Autodesk Inventor part; units mm, degrees
(part 2 of 3)
sketch "Эскиз8" plane through (0, 0, 2) normal (0, 0, 1) x (1, 0, 0)
  line L0 (83.7862, -21.9654) -> (83.7862, -32.3944) projected
  arc A0 (67.4694, -45.8121) -> (83.7862, -32.3944) centre (57.281, -16.7923) ccw projected
  line L1 (67.4694, -45.8121) -> (61.0555, -45.8121) projected
  arc A1 (53.694, -29.0439) -> (61.0555, -45.8121) centre (61.0555, -35.8121) ccw projected
  line L2 (53.694, -29.0439) -> (66.4247, -15.1972) projected
  arc A2 (83.7862, -21.9654) -> (66.4247, -15.1972) centre (73.7862, -21.9654) ccw projected
  arc A3 (-39.8825, -42.108) -> (-23.8797, -30.3072) centre (-32.521, -35.3398) ccw projected
  line L3 (-39.8825, -42.108) -> (-83.4226, 5.249) projected
  arc A4 (-86.0611, 12.0172) -> (-83.4226, 5.249) centre (-76.0611, 12.0172) ccw projected
  line L4 (-86.0611, 12.0172) -> (-86.0611, 12.0731) projected
  arc A5 (-70.312, 20.2554) -> (-86.0611, 12.0731) centre (-76.0611, 12.0731) ccw projected
  arc A6 (-23.8797, -30.3072) -> (-70.312, 20.2554) centre (-162.6046, -111.0994) ccw projected
  arc A7 (-180.9948, -7.5859) -> (-176.4785, -21.5706) centre (-134.5611, -0.3121) ccw projected
  arc A8 (-176.055, -1.8121) -> (-180.9948, -7.5859) centre (-176.055, -6.8121) ccw projected
  line L5 (-176.055, -1.8121) -> (-162.3245, -1.8121) projected
  arc A9 (-155.2534, -18.8832) -> (-162.3245, -1.8121) centre (-162.3245, -11.8121) ccw projected
  line L6 (-155.2534, -18.8832) -> (-160.4889, -24.1186) projected
  arc A10 (-176.4785, -21.5706) -> (-160.4889, -24.1186) centre (-167.5599, -17.0475) ccw projected
  arc A11 (139.56, -46.7458) -> (153.5447, -42.2296) centre (132.2862, -0.3121) ccw projected
  arc A12 (133.7862, -41.8061) -> (139.56, -46.7458) centre (138.7862, -41.8061) ccw projected
  line L7 (133.7862, -41.8061) -> (133.7862, -28.0756) projected
  arc A13 (150.8573, -21.0045) -> (133.7862, -28.0756) centre (143.7862, -28.0756) ccw projected
  line L8 (150.8573, -21.0045) -> (156.0927, -26.2399) projected
  arc A14 (153.5447, -42.2296) -> (156.0927, -26.2399) centre (149.0216, -33.311) ccw projected
  line L9 (-162.7567, 1.1879) -> (-176.5611, 1.1879) projected
  arc A15 (-181.5611, 6.1879) -> (-176.5611, 1.1879) centre (-176.5611, 6.1879) ccw projected
  line L10 (-181.5611, 6.1879) -> (-181.5611, 31.7702) projected
  arc A16 (-173.2978, 35.5585) -> (-181.5611, 31.7702) centre (-176.5611, 31.7702) ccw projected
  arc A17 (-155.2866, 17.836) -> (-173.2978, 35.5585) centre (-297.8894, -109.0766) ccw projected
  arc A18 (-162.7567, 1.1879) -> (-155.2866, 17.836) centre (-162.7567, 11.1879) ccw projected
  line L11 (81.1477, 5.249) -> (37.6077, -42.108) projected
  arc A19 (21.6048, -30.3072) -> (37.6077, -42.108) centre (30.2462, -35.3398) ccw projected
  arc A20 (68.0372, 20.2554) -> (21.6048, -30.3072) centre (160.3298, -111.0994) ccw projected
  arc A21 (83.7862, 12.0731) -> (68.0372, 20.2554) centre (73.7862, 12.0731) ccw projected
  line L12 (83.7862, 12.0731) -> (83.7862, 12.0172) projected
  arc A22 (81.1477, 5.249) -> (83.7862, 12.0172) centre (73.7862, 12.0172) ccw projected
  arc A23 (136.3136, 14.1371) -> (128.2552, 14.1361) centre (132.2862, -0.3121) ccw projected
  arc A24 (119.19, 16.0661) -> (128.2552, 14.1361) centre (125.5679, 23.7682) ccw projected
  arc A25 (96.4037, 38.427) -> (119.19, 16.0661) centre (240.0147, 161.9803) ccw projected
  arc A26 (100.194, 46.6879) -> (96.4037, 38.427) centre (100.194, 41.6879) ccw projected
  line L13 (100.194, 46.6879) -> (164.3686, 46.6879) projected
  arc A27 (168.1568, 38.4246) -> (164.3686, 46.6879) centre (164.3686, 41.6879) ccw projected
  arc A28 (145.382, 16.0725) -> (168.1568, 38.4246) centre (23.5217, 163.0162) ccw projected
  arc A29 (136.3136, 14.1371) -> (145.382, 16.0725) centre (138.9985, 23.7699) ccw projected
  line L14 (9.0433, 33.3984) -> (33.8141, 6.4561) projected
  arc A30 (33.8141, -7.0803) -> (33.8141, 6.4561) centre (26.4526, -0.3121) ccw projected
  line L15 (33.8141, -7.0803) -> (9.0433, -34.0226) projected
  arc A31 (0.3626, -30.6385) -> (9.0433, -34.0226) centre (5.3626, -30.6385) ccw projected
  line L16 (0.3626, -30.6385) -> (0.3626, 30.0143) projected
  arc A32 (9.0433, 33.3984) -> (0.3626, 30.0143) centre (5.3626, 30.0143) ccw projected
  arc A33 (-166.6434, 46.6879) -> (-170.4316, 38.4246) centre (-166.6434, 41.6879) ccw projected
  line L17 (-166.6434, 46.6879) -> (-102.4688, 46.6879) projected
  arc A34 (-98.6785, 38.427) -> (-102.4688, 46.6879) centre (-102.4688, 41.6879) ccw projected
  arc A35 (-121.4649, 16.0661) -> (-98.6785, 38.427) centre (-242.2895, 161.9803) ccw projected
  arc A36 (-130.53, 14.1361) -> (-121.4649, 16.0661) centre (-127.8427, 23.7682) ccw projected
  arc A37 (-130.53, 14.1361) -> (-138.5884, 14.1371) centre (-134.5611, -0.3121) ccw projected
  arc A38 (-147.6568, 16.0725) -> (-138.5884, 14.1371) centre (-141.2733, 23.7699) ccw projected
  arc A39 (-170.4316, 38.4246) -> (-147.6568, 16.0725) centre (-25.7966, 163.0162) ccw projected
  line L18 (-68.6995, -15.1972) -> (-55.9689, -29.0439) projected
  arc A40 (-63.3304, -45.8121) -> (-55.9689, -29.0439) centre (-63.3304, -35.8121) ccw projected
  line L19 (-63.3304, -45.8121) -> (-69.7443, -45.8121) projected
  arc A41 (-86.0611, -32.3944) -> (-69.7443, -45.8121) centre (-59.5558, -16.7923) ccw projected
  line L20 (-86.0611, -32.3944) -> (-86.0611, -21.9654) projected
  arc A42 (-68.6995, -15.1972) -> (-86.0611, -21.9654) centre (-76.0611, -21.9654) ccw projected
  line L21 (158.214, -24.1186) -> (152.9786, -18.8832) projected
  arc A43 (160.0497, -1.8121) -> (152.9786, -18.8832) centre (160.0497, -11.8121) ccw projected
  line L22 (160.0497, -1.8121) -> (173.7802, -1.8121) projected
  arc A44 (178.72, -7.5859) -> (173.7802, -1.8121) centre (173.7802, -6.8121) ccw projected
  arc A45 (174.2037, -21.5706) -> (178.72, -7.5859) centre (132.2862, -0.3121) ccw projected
  arc A46 (158.214, -24.1186) -> (174.2037, -21.5706) centre (165.2851, -17.0475) ccw projected
  arc A47 (95.0878, 34.2305) -> (86.7862, 30.4755) centre (91.7862, 30.4755) ccw projected
  arc A48 (115.908, 12.7841) -> (95.0878, 34.2305) centre (-30.0061, -108.0406) ccw projected
  arc A49 (117.838, 3.7189) -> (115.908, 12.7841) centre (108.2059, 6.4063) ccw projected
  arc A50 (117.838, 3.7189) -> (117.837, -4.3395) centre (132.2862, -0.3121) ccw projected
  arc A51 (115.9016, -13.4079) -> (117.837, -4.3395) centre (108.2042, -7.0244) ccw projected
  arc A52 (95.0899, -34.8414) -> (115.9016, -13.4079) centre (-31.0421, 108.4524) ccw projected
  arc A53 (86.7862, -31.0883) -> (95.0899, -34.8414) centre (91.7862, -31.0883) ccw projected
  line L23 (86.7862, -31.0883) -> (86.7862, 30.4755) projected
  arc A54 (174.2862, 1.1879) -> (179.2862, 6.1879) centre (174.2862, 6.1879) ccw projected
  line L24 (174.2862, 1.1879) -> (160.4818, 1.1879) projected
  arc A55 (153.0118, 17.836) -> (160.4818, 1.1879) centre (160.4818, 11.1879) ccw projected
  arc A56 (171.0229, 35.5585) -> (153.0118, 17.836) centre (295.6146, -109.0766) ccw projected
  arc A57 (179.2862, 31.7702) -> (171.0229, 35.5585) centre (174.2862, 31.7702) ccw projected
  line L25 (179.2862, 31.7702) -> (179.2862, 6.1879) projected
  line L26 (-11.3182, -34.0226) -> (-36.0889, -7.0803) projected
  arc A58 (-36.0889, 6.4561) -> (-36.0889, -7.0803) centre (-28.7274, -0.3121) ccw projected
  line L27 (-36.0889, 6.4561) -> (-11.3182, 33.3984) projected
  arc A59 (-2.6374, 30.0143) -> (-11.3182, 33.3984) centre (-7.6374, 30.0143) ccw projected
  line L28 (-2.6374, 30.0143) -> (-2.6374, -30.6385) projected
  arc A60 (-11.3182, -34.0226) -> (-2.6374, -30.6385) centre (-7.6374, -30.6385) ccw projected
  line L29 (-158.3675, -26.2399) -> (-153.1321, -21.0045) projected
  arc A61 (-136.0611, -28.0756) -> (-153.1321, -21.0045) centre (-146.0611, -28.0756) ccw projected
  line L30 (-136.0611, -28.0756) -> (-136.0611, -41.8061) projected
  arc A62 (-141.8349, -46.7458) -> (-136.0611, -41.8061) centre (-141.0611, -41.8061) ccw projected
  arc A63 (-155.8196, -42.2296) -> (-141.8349, -46.7458) centre (-134.5611, -0.3121) ccw projected
  arc A64 (-158.3675, -26.2399) -> (-155.8196, -42.2296) centre (-151.2965, -33.311) ccw projected
  arc A65 (-120.1118, -4.3395) -> (-120.1128, 3.7189) centre (-134.5611, -0.3121) ccw projected
  arc A66 (-118.1829, 12.7841) -> (-120.1128, 3.7189) centre (-110.4807, 6.4063) ccw projected
  arc A67 (-97.3626, 34.2305) -> (-118.1829, 12.7841) centre (27.7313, -108.0406) ccw projected
  arc A68 (-89.0611, 30.4755) -> (-97.3626, 34.2305) centre (-94.0611, 30.4755) ccw projected
  line L31 (-89.0611, 30.4755) -> (-89.0611, -31.0883) projected
  arc A69 (-97.3647, -34.8414) -> (-89.0611, -31.0883) centre (-94.0611, -31.0883) ccw projected
  arc A70 (-118.1765, -13.4079) -> (-97.3647, -34.8414) centre (28.7673, 108.4524) ccw projected
  arc A71 (-120.1118, -4.3395) -> (-118.1765, -13.4079) centre (-110.479, -7.0244) ccw projected
  arc A72 (-102.4787, -47.3121) -> (-98.6905, -39.0488) centre (-102.4787, -42.3121) ccw projected
  line L32 (-102.4787, -47.3121) -> (-128.0611, -47.3121) projected
  arc A73 (-133.0611, -42.3121) -> (-128.0611, -47.3121) centre (-128.0611, -42.3121) ccw projected
  line L33 (-133.0611, -42.3121) -> (-133.0611, -28.5077) projected
  arc A74 (-116.4129, -21.0376) -> (-133.0611, -28.5077) centre (-123.0611, -28.5077) ccw projected
  arc A75 (-98.6905, -39.0488) -> (-116.4129, -21.0376) centre (-243.3255, -163.6405) ccw projected
  arc A76 (-74.1343, 46.6879) -> (-77.8151, 38.3038) centre (-74.1343, 41.6879) ccw projected
  line L34 (-74.1343, 46.6879) -> (-14.5641, 46.6879) projected
  arc A77 (-10.8834, 38.3038) -> (-14.5641, 46.6879) centre (-14.5641, 41.6879) ccw projected
  line L35 (-10.8834, 38.3038) -> (-36.9877, 9.911) projected
  arc A78 (-51.7107, 9.911) -> (-36.9877, 9.911) centre (-44.3492, 16.6792) ccw projected
  line L36 (-51.7107, 9.911) -> (-77.8151, 38.3038) projected
  arc A79 (130.7862, -28.5077) -> (114.1381, -21.0376) centre (120.7862, -28.5077) ccw projected
  line L37 (130.7862, -28.5077) -> (130.7862, -42.3121) projected
  arc A80 (125.7862, -47.3121) -> (130.7862, -42.3121) centre (125.7862, -42.3121) ccw projected
  line L38 (125.7862, -47.3121) -> (100.2039, -47.3121) projected
  arc A81 (96.4156, -39.0488) -> (100.2039, -47.3121) centre (100.2039, -42.3121) ccw projected
  arc A82 (114.1381, -21.0376) -> (96.4156, -39.0488) centre (241.0507, -163.6405) ccw projected
  line L39 (75.5403, 38.3038) -> (49.4359, 9.911) projected
  arc A83 (34.7129, 9.911) -> (49.4359, 9.911) centre (42.0744, 16.6792) ccw projected
  line L40 (34.7129, 9.911) -> (8.6085, 38.3038) projected
  arc A84 (12.2893, 46.6879) -> (8.6085, 38.3038) centre (12.2893, 41.6879) ccw projected
  line L41 (12.2893, 46.6879) -> (71.8595, 46.6879) projected
  arc A85 (75.5403, 38.3038) -> (71.8595, 46.6879) centre (71.8595, 41.6879) ccw projected
  line L42 (179.2862, 51.6879) -> (-181.5611, 51.6879) projected
  arc A86 (-181.5611, 51.6879) -> (-186.5611, 46.6879) centre (-181.5611, 46.6879) ccw projected
  line L43 (-186.5611, 46.6879) -> (-186.5611, -0.3121) projected
  arc A87 (-186.5611, -0.3121) -> (-134.5611, -52.3121) centre (-134.5611, -0.3121) ccw projected
  line L44 (-134.5611, -52.3121) -> (132.2862, -52.3121) projected
  arc A88 (132.2862, -52.3121) -> (184.2862, -0.3121) centre (132.2862, -0.3121) ccw projected
  line L45 (184.2862, -0.3121) -> (184.2862, 46.6879) projected
  arc A89 (184.2862, 46.6879) -> (179.2862, 51.6879) centre (179.2862, 46.6879) ccw projected
  circle A90 centre (85.2862, -47.3121) radius 2.1 projected
  circle A91 centre (179.2862, 46.6879) radius 2.1 projected
  circle A92 centre (85.2862, 46.6879) radius 2.1 projected
  circle A93 centre (-1.1374, 46.6879) radius 2.1 projected
  circle A94 centre (-87.5611, 46.6879) radius 2.1 projected
  circle A95 centre (-181.5611, 46.6879) radius 2.1 projected
  circle A96 centre (-87.5611, -47.3121) radius 2.1 projected
  circle A97 centre (123.2862, -0.3121) radius 2.1 projected
  circle A98 centre (132.2862, 8.6879) radius 2.1 projected
  circle A99 centre (-125.5611, -0.3121) radius 2.1 projected
  circle A100 centre (-134.5611, -9.3121) radius 2.1 projected
  circle A101 centre (-134.5611, 8.6879) radius 2.1 projected
  circle A102 centre (-1.1374, -47.3121) radius 2.1 projected
  circle A103 centre (132.2862, -0.3121) radius 4 projected
  circle A104 centre (132.2862, -9.3121) radius 2.1 projected
  circle A105 centre (141.2862, -0.3121) radius 2.1 projected
  circle A106 centre (-143.5611, -0.3121) radius 2.1 projected
  circle A107 centre (-134.5611, -0.3121) radius 4 projected
  line L46 (132.2862, -47.3121) -> (-134.5611, -47.3121)
  arc A108 (-181.5611, -0.3121) -> (-134.5611, -47.3121) centre (-134.5611, -0.3121) ccw
  line L47 (-181.5611, -0.3121) -> (-181.5611, 46.6879)
  line L48 (-181.5611, 46.6879) -> (179.2862, 46.6879)
  line L49 (179.2862, 46.6879) -> (179.2862, -0.3121)
  arc A109 (132.2862, -47.3121) -> (179.2862, -0.3121) centre (132.2862, -0.3121) ccw
  line L50 (-87.5611, -52.3121) -> (-87.5611, -33.3121)
  line L51 (-87.5611, -33.3121) -> (-207.6837, -33.3121)
  line L52 (-207.6837, -33.3121) -> (179.2862, -33.3121)
  point P0 (0, 0)
  point P1 (-174.7481, -33.3121)
  point P2 (172.4733, -33.3121)
  point P3 (153.3812, -42.3121)
  point P4 (133.8119, -42.3121)
  point P5 (95.2039, -42.3121)
  point P6 (83.2242, -33.3121)
  point P7 (51.3731, -33.3121)
  point P8 (37.4147, -42.3121)
  point P9 (20.4539, -33.3121)
  point P10 (-22.7287, -33.3121)
  point P11 (-39.6895, -42.3121)
  point P12 (-53.6479, -33.3121)
  point P13 (-85.499, -33.3121)
  point P14 (130.7862, -33.3121)
  point P15 (101.5627, -33.3121)
  point P16 (159.0216, -33.3121)
  point P17 (133.7862, -33.3121)
  point P18 (45.6946, -33.3121)
  point P19 (-47.9694, -33.3121)
  dimension "d101" = 19
  constraints: 12 end point, 4 point on circle, 2 centre point, 2 perpendicular, 2 point on line, 8 other
  measures "d101" distance of L50.start L50.end
extrude "Выдавливание6" cut sketch "Эскиз8" against normal blind 2 contours L52 A53 A52 A82 A81 L46 A90 A102 A96 L50 A41 L19 A40 L3 A3 L26 A60 A31 L15 A19 L11 A1 L1 A0 | A0 L1 A1 L52 | L52 A52 A53 | L11 A19 L52 | L52 L37 A80 L38 A81 A82 | L15 A31 L52 | L52 L7 A12 A109 L46 A80 L37 | L38 L46 A109 A11 L52 A88 L44 L50 A96 A102 A90 | L52 A14 A11 A12 L7 | A60 L26 L52 | L52 A109 A14 | A3 L3 L52 | A40 L19 A41 L52 | L44 A87 L51 A108 A63 L46 L32 A96 L50 | A96 L46 A72 A75 L51 A70 A69 L50 | A69 A70 L51 | L32 A73 L33 L51 A75 A72 | L51 A64 A108 | L46 A108 A62 L30 L51 L33 A73 | A64 L51 L30 A62 A63
sketch "Эскиз9" plane through (0, 0, 2) normal (0, 0, 1) x (1, 0, 0)
  arc A0 (-186.5611, -0.3121) -> (-174.7481, -33.3121) centre (-134.5611, -0.3121) ccw projected
  arc A1 (172.4733, -33.3121) -> (184.2862, -0.3121) centre (132.2862, -0.3121) ccw projected
  line L0 (-198, -37.3121) -> (220, -37.3121)
  line L1 (-198, -28.3121) -> (220, -28.3121)
  line L2 (-174.7481, -33.3121) -> (-161.2965, -33.3121) projected
  line L3 (-174.7481, -33.3121) -> (172.4733, -33.3121)
  point P0 (0, 0)
  point P1 (168.8239, -37.3121)
  point P2 (-171.0987, -37.3121)
  point P3 (176.104, -28.3121)
  point P4 (-178.3789, -28.3121)
  dimension "d118" = 9
  constraints: 6 end point, 1 collinear, 1 parallel
  measures "d118" distance between parallel lines of L0 L1
extrude "Выдавливание7" add sketch "Эскиз9" against normal blind 2
fillet "Сопряжение6" radius 3 26 edges at (-174.7481, -33.3121, 1) (172.4733, -33.3121, 1) (-159.9574, -28.3121, 1) (-136.0611, -28.3121, 1) (-133.0592, -28.3121, 1) (-108.683, -28.3121, 1) (-104.4163, -28.3121, 1) (-89.0611, -28.3121, 1) (-86.0611, -28.3121, 1) (-56.6417, -28.3121, 1) (-25.061, -28.3121, 1) (-2.6374, -28.3121, 1) (14.2936, -28.3121, 1) (50.2916, -28.3121, 1) (83.7862, -28.3121, 1) (102.1414, -28.3121, 1) (130.7843, -28.3121, 1) (157.6826, -28.3121, 1) (-52.5665, -28.3121, 1) (-16.5684, -28.3121, 1) (0.3626, -28.3121, 1) (22.7861, -28.3121, 1) (54.3669, -28.3121, 1) (86.7862, -28.3121, 1) (106.4081, -28.3121, 1) (133.7862, -28.3121, 1)
sketch "Эскиз10" plane through (0, 0, 2) normal (0, 0, 1) x (1, 0, 0)
  circle A0 centre (-87.5611, 46.6879) radius 2.1 projected
  circle A1 centre (-1.1374, 46.6879) radius 2.1 projected
  circle A2 centre (85.2862, 46.6879) radius 2.1 projected
  line L0 (179.2862, 51.6879) -> (-181.5611, 51.6879) projected
  line L1 (-1.1374, 51.6879) -> (-1.1374, -33.3121)
  line L2 (171.029, -33.3121) -> (-173.3038, -33.3121) projected
  line L3 (-1.1374, 9.1879) -> (-298, 9.1879)
  line L4 (-298, 9.1879) -> (290, 9.1879)
  circle A3 centre (-87.5611, -28.3121) radius 2.1
  circle A4 centre (-1.1374, -28.3121) radius 2.1
  circle A5 centre (85.2862, -28.3121) radius 2.1
  point P0 (0, 0)
  constraints: 6 end point, 3 centre point, 3 midpoint, 3 symmetric about line, 2 horizontal, 3 other
extrude "Выдавливание8" cut sketch "Эскиз10" against normal blind 2 contours A4 L1 | L1 A4 | A3 | A5
sketch "Эскиз11" plane through (0, 0, 2) normal (0, 0, 1) x (1, 0, 0)
  arc A0 (171.029, -33.3121) -> (173.401, -32.1488) centre (171.029, -30.3121) ccw projected
  arc A1 (173.401, -32.1488) -> (184.2862, -0.3121) centre (132.2862, -0.3121) ccw projected
  line L0 (184.2862, -0.3121) -> (184.2862, 46.6879) projected
  arc A2 (184.2862, 46.6879) -> (179.2862, 51.6879) centre (179.2862, 46.6879) ccw projected
  line L1 (179.2862, 51.6879) -> (-181.5611, 51.6879) projected
  arc A3 (-181.5611, 51.6879) -> (-186.5611, 46.6879) centre (-181.5611, 46.6879) ccw projected
  line L2 (-186.5611, 46.6879) -> (-186.5611, -0.3121) projected
  arc A4 (-186.5611, -0.3121) -> (-175.6758, -32.1488) centre (-134.5611, -0.3121) ccw projected
  arc A5 (-175.6758, -32.1488) -> (-173.3038, -33.3121) centre (-173.3038, -30.3121) ccw projected
  line L3 (-173.3038, -33.3121) -> (171.029, -33.3121) projected
  line L4 (-155.3184, -23.1908) -> (-153.1321, -21.0045) projected
  arc A6 (-136.8733, -24.1278) -> (-153.1321, -21.0045) centre (-146.0611, -28.0756) ccw projected
  arc A7 (68.0372, 20.2554) -> (25.6837, -23.6784) centre (160.3298, -111.0994) ccw projected
  arc A8 (83.7862, 12.0731) -> (68.0372, 20.2554) centre (73.7862, 12.0731) ccw projected
  line L5 (83.7862, 12.0731) -> (83.7862, 12.0172) projected
  arc A9 (81.1477, 5.249) -> (83.7862, 12.0172) centre (73.7862, 12.0172) ccw projected
  line L6 (81.1477, 5.249) -> (51.183, -27.3426) projected
  line L7 (-53.4579, -27.3426) -> (-83.4226, 5.249) projected
  arc A10 (-86.0611, 12.0172) -> (-83.4226, 5.249) centre (-76.0611, 12.0172) ccw projected
  line L8 (-86.0611, 12.0172) -> (-86.0611, 12.0731) projected
  arc A11 (-70.312, 20.2554) -> (-86.0611, 12.0731) centre (-76.0611, 12.0731) ccw projected
  arc A12 (-27.9585, -23.6784) -> (-70.312, 20.2554) centre (-162.6046, -111.0994) ccw projected
  arc A13 (114.1381, -21.0376) -> (111.8541, -23.1036) centre (241.0507, -163.6405) ccw projected
  arc A14 (129.6834, -23.9426) -> (114.1381, -21.0376) centre (120.7862, -28.5077) ccw projected
  arc A15 (-68.6995, -15.1972) -> (-86.0611, -21.9654) centre (-76.0611, -21.9654) ccw projected
  line L9 (-68.6995, -15.1972) -> (-61.2667, -23.2817) projected
  line L10 (58.9919, -23.2817) -> (66.4247, -15.1972) projected
  arc A16 (83.7862, -21.9654) -> (66.4247, -15.1972) centre (73.7862, -21.9654) ccw projected
  line L11 (83.7862, -21.9654) -> (83.7862, -25.3121) projected
  arc A17 (-116.4129, -21.0376) -> (-131.9582, -23.9426) centre (-123.0611, -28.5077) ccw projected
  arc A18 (-114.1289, -23.1036) -> (-116.4129, -21.0376) centre (-243.3255, -163.6405) ccw projected
  arc A19 (150.8573, -21.0045) -> (134.5985, -24.1278) centre (143.7862, -28.0756) ccw projected
  line L12 (150.8573, -21.0045) -> (153.0436, -23.1908) projected
  circle A20 centre (-134.5611, -0.3121) radius 4 projected
  circle A21 centre (-143.5611, -0.3121) radius 2.1 projected
  circle A22 centre (141.2862, -0.3121) radius 2.1 projected
  circle A23 centre (132.2862, -9.3121) radius 2.1 projected
  circle A24 centre (132.2862, -0.3121) radius 4 projected
  circle A25 centre (-134.5611, 8.6879) radius 2.1 projected
  circle A26 centre (-134.5611, -9.3121) radius 2.1 projected
  circle A27 centre (-125.5611, -0.3121) radius 2.1 projected
  circle A28 centre (132.2862, 8.6879) radius 2.1 projected
  circle A29 centre (123.2862, -0.3121) radius 2.1 projected
  circle A30 centre (-181.5611, 46.6879) radius 2.1 projected
  circle A31 centre (-87.5611, 46.6879) radius 2.1 projected
  circle A32 centre (-1.1374, 46.6879) radius 2.1 projected
  circle A33 centre (85.2862, 46.6879) radius 2.1 projected
  circle A34 centre (179.2862, 46.6879) radius 2.1 projected
  line L13 (75.5403, 38.3038) -> (49.4359, 9.911) projected
  arc A35 (34.7129, 9.911) -> (49.4359, 9.911) centre (42.0744, 16.6792) ccw projected
  line L14 (34.7129, 9.911) -> (8.6085, 38.3038) projected
  arc A36 (12.2893, 46.6879) -> (8.6085, 38.3038) centre (12.2893, 41.6879) ccw projected
  line L15 (12.2893, 46.6879) -> (71.8595, 46.6879) projected
  arc A37 (75.5403, 38.3038) -> (71.8595, 46.6879) centre (71.8595, 41.6879) ccw projected
  arc A38 (-74.1343, 46.6879) -> (-77.8151, 38.3038) centre (-74.1343, 41.6879) ccw projected
  line L16 (-74.1343, 46.6879) -> (-14.5641, 46.6879) projected
  arc A39 (-10.8834, 38.3038) -> (-14.5641, 46.6879) centre (-14.5641, 41.6879) ccw projected
  line L17 (-10.8834, 38.3038) -> (-36.9877, 9.911) projected
  arc A40 (-51.7107, 9.911) -> (-36.9877, 9.911) centre (-44.3492, 16.6792) ccw projected
  line L18 (-51.7107, 9.911) -> (-77.8151, 38.3038) projected
  arc A41 (-120.1118, -4.3395) -> (-120.1128, 3.7189) centre (-134.5611, -0.3121) ccw projected
  arc A42 (-118.1829, 12.7841) -> (-120.1128, 3.7189) centre (-110.4807, 6.4063) ccw projected
  arc A43 (-97.3626, 34.2305) -> (-118.1829, 12.7841) centre (27.7313, -108.0406) ccw projected
  arc A44 (-89.0611, 30.4755) -> (-97.3626, 34.2305) centre (-94.0611, 30.4755) ccw projected
  line L19 (-89.0611, 30.4755) -> (-89.0611, -25.3121) projected
  arc A45 (-118.1765, -13.4079) -> (-105.2981, -27.4478) centre (28.7673, 108.4524) ccw projected
  arc A46 (-120.1118, -4.3395) -> (-118.1765, -13.4079) centre (-110.479, -7.0244) ccw projected
  line L20 (-17.4598, -27.3426) -> (-36.0889, -7.0803) projected
  arc A47 (-36.0889, 6.4561) -> (-36.0889, -7.0803) centre (-28.7274, -0.3121) ccw projected
  line L21 (-36.0889, 6.4561) -> (-11.3182, 33.3984) projected
  arc A48 (-2.6374, 30.0143) -> (-11.3182, 33.3984) centre (-7.6374, 30.0143) ccw projected
  line L22 (-2.6374, 30.0143) -> (-2.6374, -25.3121) projected
  arc A49 (174.2862, 1.1879) -> (179.2862, 6.1879) centre (174.2862, 6.1879) ccw projected
  line L23 (174.2862, 1.1879) -> (160.4818, 1.1879) projected
  arc A50 (153.0118, 17.836) -> (160.4818, 1.1879) centre (160.4818, 11.1879) ccw projected
  arc A51 (171.0229, 35.5585) -> (153.0118, 17.836) centre (295.6146, -109.0766) ccw projected
  arc A52 (179.2862, 31.7702) -> (171.0229, 35.5585) centre (174.2862, 31.7702) ccw projected
  line L24 (179.2862, 31.7702) -> (179.2862, 6.1879) projected
  arc A53 (95.0878, 34.2305) -> (86.7862, 30.4755) centre (91.7862, 30.4755) ccw projected
  arc A54 (115.908, 12.7841) -> (95.0878, 34.2305) centre (-30.0061, -108.0406) ccw projected
  arc A55 (117.838, 3.7189) -> (115.908, 12.7841) centre (108.2059, 6.4063) ccw projected
  arc A56 (117.838, 3.7189) -> (117.837, -4.3395) centre (132.2862, -0.3121) ccw projected
  arc A57 (115.9016, -13.4079) -> (117.837, -4.3395) centre (108.2042, -7.0244) ccw projected
  arc A58 (103.0232, -27.4478) -> (115.9016, -13.4079) centre (-31.0421, 108.4524) ccw projected
  line L25 (86.7862, -25.3121) -> (86.7862, 30.4755) projected
  line L26 (158.214, -24.1186) -> (152.9786, -18.8832) projected
  arc A59 (160.0497, -1.8121) -> (152.9786, -18.8832) centre (160.0497, -11.8121) ccw projected
  line L27 (160.0497, -1.8121) -> (173.7802, -1.8121) projected
  arc A60 (178.72, -7.5859) -> (173.7802, -1.8121) centre (173.7802, -6.8121) ccw projected
  arc A61 (174.2037, -21.5706) -> (178.72, -7.5859) centre (132.2862, -0.3121) ccw projected
  arc A62 (158.214, -24.1186) -> (174.2037, -21.5706) centre (165.2851, -17.0475) ccw projected
  arc A63 (-166.6434, 46.6879) -> (-170.4316, 38.4246) centre (-166.6434, 41.6879) ccw projected
  line L28 (-166.6434, 46.6879) -> (-102.4688, 46.6879) projected
  arc A64 (-98.6785, 38.427) -> (-102.4688, 46.6879) centre (-102.4688, 41.6879) ccw projected
  arc A65 (-121.4649, 16.0661) -> (-98.6785, 38.427) centre (-242.2895, 161.9803) ccw projected
  arc A66 (-130.53, 14.1361) -> (-121.4649, 16.0661) centre (-127.8427, 23.7682) ccw projected
  arc A67 (-130.53, 14.1361) -> (-138.5884, 14.1371) centre (-134.5611, -0.3121) ccw projected
  arc A68 (-147.6568, 16.0725) -> (-138.5884, 14.1371) centre (-141.2733, 23.7699) ccw projected
  arc A69 (-170.4316, 38.4246) -> (-147.6568, 16.0725) centre (-25.7966, 163.0162) ccw projected
  line L29 (9.0433, 33.3984) -> (33.8141, 6.4561) projected
  arc A70 (33.8141, -7.0803) -> (33.8141, 6.4561) centre (26.4526, -0.3121) ccw projected
  line L30 (33.8141, -7.0803) -> (15.185, -27.3426) projected
  line L31 (0.3626, -25.3121) -> (0.3626, 30.0143) projected
  arc A71 (9.0433, 33.3984) -> (0.3626, 30.0143) centre (5.3626, 30.0143) ccw projected
  arc A72 (136.3136, 14.1371) -> (128.2552, 14.1361) centre (132.2862, -0.3121) ccw projected
  arc A73 (119.19, 16.0661) -> (128.2552, 14.1361) centre (125.5679, 23.7682) ccw projected
  arc A74 (96.4037, 38.427) -> (119.19, 16.0661) centre (240.0147, 161.9803) ccw projected
  arc A75 (100.194, 46.6879) -> (96.4037, 38.427) centre (100.194, 41.6879) ccw projected
  line L32 (100.194, 46.6879) -> (164.3686, 46.6879) projected
  arc A76 (168.1568, 38.4246) -> (164.3686, 46.6879) centre (164.3686, 41.6879) ccw projected
  arc A77 (145.382, 16.0725) -> (168.1568, 38.4246) centre (23.5217, 163.0162) ccw projected
  arc A78 (136.3136, 14.1371) -> (145.382, 16.0725) centre (138.9985, 23.7699) ccw projected
  line L33 (-162.7567, 1.1879) -> (-176.5611, 1.1879) projected
  arc A79 (-181.5611, 6.1879) -> (-176.5611, 1.1879) centre (-176.5611, 6.1879) ccw projected
  line L34 (-181.5611, 6.1879) -> (-181.5611, 31.7702) projected
  arc A80 (-173.2978, 35.5585) -> (-181.5611, 31.7702) centre (-176.5611, 31.7702) ccw projected
  arc A81 (-155.2866, 17.836) -> (-173.2978, 35.5585) centre (-297.8894, -109.0766) ccw projected
  arc A82 (-162.7567, 1.1879) -> (-155.2866, 17.836) centre (-162.7567, 11.1879) ccw projected
  arc A83 (-180.9948, -7.5859) -> (-176.4785, -21.5706) centre (-134.5611, -0.3121) ccw projected
  arc A84 (-176.055, -1.8121) -> (-180.9948, -7.5859) centre (-176.055, -6.8121) ccw projected
  line L35 (-176.055, -1.8121) -> (-162.3245, -1.8121) projected
  arc A85 (-155.2534, -18.8832) -> (-162.3245, -1.8121) centre (-162.3245, -11.8121) ccw projected
  line L36 (-155.2534, -18.8832) -> (-160.4889, -24.1186) projected
  arc A86 (-176.4785, -21.5706) -> (-160.4889, -24.1186) centre (-167.5599, -17.0475) ccw projected
  circle A87 centre (-87.5611, -28.3121) radius 5
  circle A88 centre (-1.1374, -28.3121) radius 5
  circle A89 centre (85.2862, -28.3121) radius 5
  line L37 (-1.1374, 46.6879) -> (-1.1374, -28.3121)
  line L38 (-1.1374, 9.1879) -> (8.8626, 9.1879)
  line L39 (-2.6374, -25.3121) -> (-2.6374, 30.0143) projected
  line L40 (-1.1374, 9.1879) -> (8.8626, 9.1879) construction
  arc A90 (71.8595, -28.3121) -> (83.7862, -21.9654) centre (72.2556, -14.6768) ccw
  arc A91 (-86.0611, -21.9654) -> (-74.1343, -28.3121) centre (-74.5305, -14.6768) ccw
  circle A92 centre (85.2862, -28.3121) radius 2.1 projected
  circle A93 centre (-87.5611, -28.3121) radius 2.1 projected
  line L41 (-86.0611, -25.3121) -> (-86.0611, -21.9654) projected
  circle A94 centre (-1.1374, -28.3121) radius 2.1 projected
  line L42 (-92.0611, -28.3121) -> (-103.1912, -28.3121) projected
  line L43 (-63.4752, -28.3121) -> (-83.0611, -28.3121) projected
  line L44 (-5.6374, -28.3121) -> (-15.2513, -28.3121) projected
  line L45 (100.9164, -28.3121) -> (89.7862, -28.3121) projected
  line L46 (12.9765, -28.3121) -> (3.3626, -28.3121) projected
  line L47 (80.7862, -28.3121) -> (61.2003, -28.3121) projected
  line L48 (127.0142, -28.3121) -> (113.8844, -28.3121) projected
  line L49 (48.9746, -28.3121) -> (28.1999, -28.3121) projected
  line L50 (150.9223, -28.3121) -> (137.3548, -28.3121) projected
  line L51 (-30.4747, -28.3121) -> (-51.2494, -28.3121) projected
  line L52 (-139.6296, -28.3121) -> (-153.1971, -28.3121) projected
  line L53 (-116.1593, -28.3121) -> (-129.2891, -28.3121) projected
  arc A95 (-139.6296, -28.3121) -> (-136.8733, -24.1278) centre (-139.6296, -25.3121) ccw projected
  arc A96 (-155.3184, -23.1908) -> (-153.1971, -28.3121) centre (-153.1971, -25.3121) ccw projected
  arc A97 (100.9164, -28.3121) -> (103.0232, -27.4478) centre (100.9164, -25.3121) ccw projected
  arc A98 (127.0142, -28.3121) -> (129.6834, -23.9426) centre (127.0142, -25.3121) ccw projected
  arc A99 (80.7862, -28.3121) -> (83.7862, -25.3121) centre (80.7862, -25.3121) ccw projected
  arc A100 (48.9746, -28.3121) -> (51.183, -27.3426) centre (48.9746, -25.3121) ccw projected
  arc A101 (150.9223, -28.3121) -> (153.0436, -23.1908) centre (150.9223, -25.3121) ccw projected
  arc A102 (0.3626, -25.3121) -> (3.3626, -28.3121) centre (3.3626, -25.3121) ccw projected
  arc A103 (12.9765, -28.3121) -> (15.185, -27.3426) centre (12.9765, -25.3121) ccw projected
  arc A104 (-17.4598, -27.3426) -> (-15.2513, -28.3121) centre (-15.2513, -25.3121) ccw projected
  arc A105 (-5.6374, -28.3121) -> (-2.6374, -25.3121) centre (-5.6374, -25.3121) ccw projected
  arc A106 (-53.4579, -27.3426) -> (-51.2494, -28.3121) centre (-51.2494, -25.3121) ccw projected
  arc A107 (-30.4747, -28.3121) -> (-27.9585, -23.6784) centre (-30.4747, -25.3121) ccw projected
  arc A108 (-86.0611, -25.3121) -> (-83.0611, -28.3121) centre (-83.0611, -25.3121) ccw projected
  arc A109 (-63.4752, -28.3121) -> (-61.2667, -23.2817) centre (-63.4752, -25.3121) ccw projected
  arc A110 (-116.1593, -28.3121) -> (-114.1289, -23.1036) centre (-116.1593, -25.3121) ccw projected
  arc A111 (-131.9582, -23.9426) -> (-129.2891, -28.3121) centre (-129.2891, -25.3121) ccw projected
  arc A112 (-105.2981, -27.4478) -> (-103.1912, -28.3121) centre (-103.1912, -25.3121) ccw projected
  arc A113 (-92.0611, -28.3121) -> (-89.0611, -25.3121) centre (-92.0611, -25.3121) ccw projected
  arc A114 (86.7862, -25.3121) -> (89.7862, -28.3121) centre (89.7862, -25.3121) ccw projected
  arc A115 (111.8541, -23.1036) -> (113.8844, -28.3121) centre (113.8844, -25.3121) ccw projected
  arc A116 (58.9919, -23.2817) -> (61.2003, -28.3121) centre (61.2003, -25.3121) ccw projected
  arc A117 (25.6837, -23.6784) -> (28.1999, -28.3121) centre (28.1999, -25.3121) ccw projected
  arc A118 (134.5985, -24.1278) -> (137.3548, -28.3121) centre (137.3548, -25.3121) ccw projected
  arc A119 (86.7862, -12.0997) -> (100.194, -28.3121) centre (105.7085, -10.1012) ccw
  arc A120 (0.3626, -11.6385) -> (12.2893, -28.3121) centre (15.857, -13.1577) ccw
  arc A121 (-102.4688, -28.3121) -> (-89.0611, -12.0997) centre (-107.9833, -10.1012) ccw
  arc A122 (-14.5641, -28.3121) -> (-2.6374, -11.6385) centre (-18.1319, -13.1577) ccw
  point P0 (0, 0)
  point P1 (-2.6374, -30.6385)
  point P2 (-2.6374, -26.8424)
  point P3 (-2.6374, -26.8424)
  point P4 (72.6518, -28.3121)
  point P5 (100.194, -28.3121)
  point P6 (86.7862, -12.0997)
  point P7 (-2.6374, -14.6768)
  point P8 (-14.5641, -28.3121)
  point P9 (12.2893, -28.3121)
  point P10 (0.3626, -14.6768)
  point P11 (-74.9266, -28.3121)
  point P12 (-89.0611, -12.0997)
  point P13 (-102.4688, -28.3121)
  dimension "d110" = 10
  dimension "d111" = 10
  dimension "d112" = 10
  dimension "d113" = 10
  dimension "d114" = 0
  constraints: 13 symmetric about line, 12 point on circle, 9 centre point, 6 end point, 2 perpendicular, 1 collinear, 1 horizontal, 1 midpoint, 3 other
  measures "d110" diameter of A87
  measures "d111" diameter of A88
  measures "d112" diameter of A89
  measures "d113" distance of L38.start L38.end
  measures "d114" distance between parallel lines of L38 L40
extrude "Выдавливание9" add sketch "Эскиз11" against normal blind 2 contours L47 A90 L11 A89 | A89 L11 A99 L47 | L45 A114 L25 A89 | A89 L25 A119 L45 | L44 A122 L22 A88 | A88 L22 A105 L44 | L46 A102 L31 A88 | A88 L31 A120 L46 | L42 A121 L19 A87 | A87 L19 A113 L42 | L43 A108 L41 A87 | A87 L41 A91 L43
sketch "Эскиз13" plane through (0, 0, 0) normal (0, 0, -1) x (-1, 0, 0)
  point P0 (0, 0)
sketch "Эскиз14" plane through (0, 0, 2) normal (0, 0, 1) x (1, 0, 0)
  circle A0 centre (85.2862, -28.3121) radius 2.1 projected
  circle A1 centre (-1.1374, -28.3121) radius 2.1 projected
  circle A2 centre (-87.5611, -28.3121) radius 2.1 projected
  arc A3 (171.029, -33.3121) -> (173.401, -32.1488) centre (171.029, -30.3121) ccw projected
  arc A4 (173.401, -32.1488) -> (184.2862, -0.3121) centre (132.2862, -0.3121) ccw projected
  line L0 (184.2862, -0.3121) -> (184.2862, 46.6879) projected
  arc A5 (184.2862, 46.6879) -> (179.2862, 51.6879) centre (179.2862, 46.6879) ccw projected
  line L1 (179.2862, 51.6879) -> (-181.5611, 51.6879) projected
  arc A6 (-181.5611, 51.6879) -> (-186.5611, 46.6879) centre (-181.5611, 46.6879) ccw projected
  line L2 (-186.5611, 46.6879) -> (-186.5611, -0.3121) projected
  arc A7 (-186.5611, -0.3121) -> (-175.6758, -32.1488) centre (-134.5611, -0.3121) ccw projected
  arc A8 (-175.6758, -32.1488) -> (-173.3038, -33.3121) centre (-173.3038, -30.3121) ccw projected
  line L3 (-173.3038, -33.3121) -> (171.029, -33.3121) projected
  line L4 (86.7862, -12.0997) -> (86.7862, 30.4755) projected
  arc A9 (95.0878, 34.2305) -> (86.7862, 30.4755) centre (91.7862, 30.4755) ccw projected
  arc A10 (115.908, 12.7841) -> (95.0878, 34.2305) centre (-30.0061, -108.0406) ccw projected
  arc A11 (117.838, 3.7189) -> (115.908, 12.7841) centre (108.2059, 6.4063) ccw projected
  arc A12 (117.838, 3.7189) -> (117.837, -4.3395) centre (132.2862, -0.3121) ccw projected
  arc A13 (115.9016, -13.4079) -> (117.837, -4.3395) centre (108.2042, -7.0244) ccw projected
  arc A14 (103.0232, -27.4478) -> (115.9016, -13.4079) centre (-31.0421, 108.4524) ccw projected
  arc A15 (100.9164, -28.3121) -> (103.0232, -27.4478) centre (100.9164, -25.3121) ccw projected
  line L5 (100.9164, -28.3121) -> (100.194, -28.3121) projected
  arc A16 (86.7862, -12.0997) -> (100.194, -28.3121) centre (105.7085, -10.1012) ccw projected
  arc A17 (114.1381, -21.0376) -> (111.8541, -23.1036) centre (241.0507, -163.6405) ccw projected
  arc A18 (129.6834, -23.9426) -> (114.1381, -21.0376) centre (120.7862, -28.5077) ccw projected
  arc A19 (127.0142, -28.3121) -> (129.6834, -23.9426) centre (127.0142, -25.3121) ccw projected
  line L6 (127.0142, -28.3121) -> (113.8844, -28.3121) projected
  arc A20 (111.8541, -23.1036) -> (113.8844, -28.3121) centre (113.8844, -25.3121) ccw projected
  line L7 (72.6518, -28.3121) -> (61.2003, -28.3121) projected
  arc A21 (58.9919, -23.2817) -> (61.2003, -28.3121) centre (61.2003, -25.3121) ccw projected
  line L8 (58.9919, -23.2817) -> (66.4247, -15.1972) projected
  arc A22 (83.7862, -21.9654) -> (66.4247, -15.1972) centre (73.7862, -21.9654) ccw projected
  arc A23 (72.6518, -28.3121) -> (83.7862, -21.9654) centre (72.2556, -14.6768) ccw projected
  line L9 (48.9746, -28.3121) -> (28.1999, -28.3121) projected
  arc A24 (25.6837, -23.6784) -> (28.1999, -28.3121) centre (28.1999, -25.3121) ccw projected
  arc A25 (68.0372, 20.2554) -> (25.6837, -23.6784) centre (160.3298, -111.0994) ccw projected
  arc A26 (83.7862, 12.0731) -> (68.0372, 20.2554) centre (73.7862, 12.0731) ccw projected
  line L10 (83.7862, 12.0731) -> (83.7862, 12.0172) projected
  arc A27 (81.1477, 5.249) -> (83.7862, 12.0172) centre (73.7862, 12.0172) ccw projected
  line L11 (81.1477, 5.249) -> (51.183, -27.3426) projected
  arc A28 (48.9746, -28.3121) -> (51.183, -27.3426) centre (48.9746, -25.3121) ccw projected
  arc A29 (150.8573, -21.0045) -> (134.5985, -24.1278) centre (143.7862, -28.0756) ccw projected
  line L12 (150.8573, -21.0045) -> (153.0436, -23.1908) projected
  arc A30 (150.9223, -28.3121) -> (153.0436, -23.1908) centre (150.9223, -25.3121) ccw projected
  line L13 (150.9223, -28.3121) -> (137.3548, -28.3121) projected
  arc A31 (134.5985, -24.1278) -> (137.3548, -28.3121) centre (137.3548, -25.3121) ccw projected
  line L14 (12.9765, -28.3121) -> (12.2893, -28.3121) projected
  arc A32 (0.3626, -14.6768) -> (12.2893, -28.3121) centre (15.857, -13.1577) ccw projected
  line L15 (0.3626, -14.6768) -> (0.3626, 30.0143) projected
  arc A33 (9.0433, 33.3984) -> (0.3626, 30.0143) centre (5.3626, 30.0143) ccw projected
  line L16 (9.0433, 33.3984) -> (33.8141, 6.4561) projected
  arc A34 (33.8141, -7.0803) -> (33.8141, 6.4561) centre (26.4526, -0.3121) ccw projected
  line L17 (33.8141, -7.0803) -> (15.185, -27.3426) projected
  arc A35 (12.9765, -28.3121) -> (15.185, -27.3426) centre (12.9765, -25.3121) ccw projected
  line L18 (-14.5641, -28.3121) -> (-15.2513, -28.3121) projected
  arc A36 (-17.4598, -27.3426) -> (-15.2513, -28.3121) centre (-15.2513, -25.3121) ccw projected
  line L19 (-17.4598, -27.3426) -> (-36.0889, -7.0803) projected
  arc A37 (-36.0889, 6.4561) -> (-36.0889, -7.0803) centre (-28.7274, -0.3121) ccw projected
  line L20 (-36.0889, 6.4561) -> (-11.3182, 33.3984) projected
  arc A38 (-2.6374, 30.0143) -> (-11.3182, 33.3984) centre (-7.6374, 30.0143) ccw projected
  line L21 (-2.6374, 30.0143) -> (-2.6374, -14.6768) projected
  arc A39 (-14.5641, -28.3121) -> (-2.6374, -14.6768) centre (-18.1319, -13.1577) ccw projected
  line L22 (-30.4747, -28.3121) -> (-51.2494, -28.3121) projected
  arc A40 (-53.4579, -27.3426) -> (-51.2494, -28.3121) centre (-51.2494, -25.3121) ccw projected
  line L23 (-53.4579, -27.3426) -> (-83.4226, 5.249) projected
  arc A41 (-86.0611, 12.0172) -> (-83.4226, 5.249) centre (-76.0611, 12.0172) ccw projected
  line L24 (-86.0611, 12.0172) -> (-86.0611, 12.0731) projected
  arc A42 (-70.312, 20.2554) -> (-86.0611, 12.0731) centre (-76.0611, 12.0731) ccw projected
  arc A43 (-27.9585, -23.6784) -> (-70.312, 20.2554) centre (-162.6046, -111.0994) ccw projected
  arc A44 (-30.4747, -28.3121) -> (-27.9585, -23.6784) centre (-30.4747, -25.3121) ccw projected
  line L25 (-155.3184, -23.1908) -> (-153.1321, -21.0045) projected
  arc A45 (-136.8733, -24.1278) -> (-153.1321, -21.0045) centre (-146.0611, -28.0756) ccw projected
  arc A46 (-139.6296, -28.3121) -> (-136.8733, -24.1278) centre (-139.6296, -25.3121) ccw projected
  line L26 (-139.6296, -28.3121) -> (-153.1971, -28.3121) projected
  arc A47 (-155.3184, -23.1908) -> (-153.1971, -28.3121) centre (-153.1971, -25.3121) ccw projected
  line L27 (-63.4752, -28.3121) -> (-74.9266, -28.3121) projected
  arc A48 (-86.0611, -21.9654) -> (-74.9266, -28.3121) centre (-74.5305, -14.6768) ccw projected
  arc A49 (-68.6995, -15.1972) -> (-86.0611, -21.9654) centre (-76.0611, -21.9654) ccw projected
  line L28 (-68.6995, -15.1972) -> (-61.2667, -23.2817) projected
  arc A50 (-63.4752, -28.3121) -> (-61.2667, -23.2817) centre (-63.4752, -25.3121) ccw projected
  arc A51 (-116.4129, -21.0376) -> (-131.9582, -23.9426) centre (-123.0611, -28.5077) ccw projected
  arc A52 (-114.1289, -23.1036) -> (-116.4129, -21.0376) centre (-243.3255, -163.6405) ccw projected
  arc A53 (-116.1593, -28.3121) -> (-114.1289, -23.1036) centre (-116.1593, -25.3121) ccw projected
  line L29 (-116.1593, -28.3121) -> (-129.2891, -28.3121) projected
  arc A54 (-131.9582, -23.9426) -> (-129.2891, -28.3121) centre (-129.2891, -25.3121) ccw projected
  circle A55 centre (-134.5611, -0.3121) radius 4 projected
  circle A56 centre (-143.5611, -0.3121) radius 2.1 projected
  circle A57 centre (141.2862, -0.3121) radius 2.1 projected
  circle A58 centre (132.2862, -9.3121) radius 2.1 projected
  circle A59 centre (132.2862, -0.3121) radius 4 projected
  circle A60 centre (-134.5611, 8.6879) radius 2.1 projected
  circle A61 centre (-134.5611, -9.3121) radius 2.1 projected
  circle A62 centre (-125.5611, -0.3121) radius 2.1 projected
  circle A63 centre (132.2862, 8.6879) radius 2.1 projected
  circle A64 centre (123.2862, -0.3121) radius 2.1 projected
  circle A65 centre (-181.5611, 46.6879) radius 2.1 projected
  circle A66 centre (-87.5611, 46.6879) radius 2.1 projected
  circle A67 centre (-1.1374, 46.6879) radius 2.1 projected
  circle A68 centre (85.2862, 46.6879) radius 2.1 projected
  circle A69 centre (179.2862, 46.6879) radius 2.1 projected
  line L30 (75.5403, 38.3038) -> (49.4359, 9.911) projected
  arc A70 (34.7129, 9.911) -> (49.4359, 9.911) centre (42.0744, 16.6792) ccw projected
  line L31 (34.7129, 9.911) -> (8.6085, 38.3038) projected
  arc A71 (12.2893, 46.6879) -> (8.6085, 38.3038) centre (12.2893, 41.6879) ccw projected
  line L32 (12.2893, 46.6879) -> (71.8595, 46.6879) projected
  arc A72 (75.5403, 38.3038) -> (71.8595, 46.6879) centre (71.8595, 41.6879) ccw projected
  arc A73 (-74.1343, 46.6879) -> (-77.8151, 38.3038) centre (-74.1343, 41.6879) ccw projected
  line L33 (-74.1343, 46.6879) -> (-14.5641, 46.6879) projected
  arc A74 (-10.8834, 38.3038) -> (-14.5641, 46.6879) centre (-14.5641, 41.6879) ccw projected
  line L34 (-10.8834, 38.3038) -> (-36.9877, 9.911) projected
  arc A75 (-51.7107, 9.911) -> (-36.9877, 9.911) centre (-44.3492, 16.6792) ccw projected
  line L35 (-51.7107, 9.911) -> (-77.8151, 38.3038) projected
  arc A76 (174.2862, 1.1879) -> (179.2862, 6.1879) centre (174.2862, 6.1879) ccw projected
  line L36 (174.2862, 1.1879) -> (160.4818, 1.1879) projected
  arc A77 (153.0118, 17.836) -> (160.4818, 1.1879) centre (160.4818, 11.1879) ccw projected
  arc A78 (171.0229, 35.5585) -> (153.0118, 17.836) centre (295.6146, -109.0766) ccw projected
  arc A79 (179.2862, 31.7702) -> (171.0229, 35.5585) centre (174.2862, 31.7702) ccw projected
  line L37 (179.2862, 31.7702) -> (179.2862, 6.1879) projected
  line L38 (158.214, -24.1186) -> (152.9786, -18.8832) projected
  arc A80 (160.0497, -1.8121) -> (152.9786, -18.8832) centre (160.0497, -11.8121) ccw projected
  line L39 (160.0497, -1.8121) -> (173.7802, -1.8121) projected
  arc A81 (178.72, -7.5859) -> (173.7802, -1.8121) centre (173.7802, -6.8121) ccw projected
  arc A82 (174.2037, -21.5706) -> (178.72, -7.5859) centre (132.2862, -0.3121) ccw projected
  arc A83 (158.214, -24.1186) -> (174.2037, -21.5706) centre (165.2851, -17.0475) ccw projected
  arc A84 (-166.6434, 46.6879) -> (-170.4316, 38.4246) centre (-166.6434, 41.6879) ccw projected
  line L40 (-166.6434, 46.6879) -> (-102.4688, 46.6879) projected
  arc A85 (-98.6785, 38.427) -> (-102.4688, 46.6879) centre (-102.4688, 41.6879) ccw projected
  arc A86 (-121.4649, 16.0661) -> (-98.6785, 38.427) centre (-242.2895, 161.9803) ccw projected
  arc A87 (-130.53, 14.1361) -> (-121.4649, 16.0661) centre (-127.8427, 23.7682) ccw projected
  arc A88 (-130.53, 14.1361) -> (-138.5884, 14.1371) centre (-134.5611, -0.3121) ccw projected
  arc A89 (-147.6568, 16.0725) -> (-138.5884, 14.1371) centre (-141.2733, 23.7699) ccw projected
  arc A90 (-170.4316, 38.4246) -> (-147.6568, 16.0725) centre (-25.7966, 163.0162) ccw projected
  arc A91 (136.3136, 14.1371) -> (128.2552, 14.1361) centre (132.2862, -0.3121) ccw projected
  arc A92 (119.19, 16.0661) -> (128.2552, 14.1361) centre (125.5679, 23.7682) ccw projected
  arc A93 (96.4037, 38.427) -> (119.19, 16.0661) centre (240.0147, 161.9803) ccw projected
  arc A94 (100.194, 46.6879) -> (96.4037, 38.427) centre (100.194, 41.6879) ccw projected
  line L41 (100.194, 46.6879) -> (164.3686, 46.6879) projected
  arc A95 (168.1568, 38.4246) -> (164.3686, 46.6879) centre (164.3686, 41.6879) ccw projected
  arc A96 (145.382, 16.0725) -> (168.1568, 38.4246) centre (23.5217, 163.0162) ccw projected
  arc A97 (136.3136, 14.1371) -> (145.382, 16.0725) centre (138.9985, 23.7699) ccw projected
  line L42 (-162.7567, 1.1879) -> (-176.5611, 1.1879) projected
  arc A98 (-181.5611, 6.1879) -> (-176.5611, 1.1879) centre (-176.5611, 6.1879) ccw projected
  line L43 (-181.5611, 6.1879) -> (-181.5611, 31.7702) projected
  arc A99 (-173.2978, 35.5585) -> (-181.5611, 31.7702) centre (-176.5611, 31.7702) ccw projected
  arc A100 (-155.2866, 17.836) -> (-173.2978, 35.5585) centre (-297.8894, -109.0766) ccw projected
  arc A101 (-162.7567, 1.1879) -> (-155.2866, 17.836) centre (-162.7567, 11.1879) ccw projected
  arc A102 (-180.9948, -7.5859) -> (-176.4785, -21.5706) centre (-134.5611, -0.3121) ccw projected
  arc A103 (-176.055, -1.8121) -> (-180.9948, -7.5859) centre (-176.055, -6.8121) ccw projected
  line L44 (-176.055, -1.8121) -> (-162.3245, -1.8121) projected
  arc A104 (-155.2534, -18.8832) -> (-162.3245, -1.8121) centre (-162.3245, -11.8121) ccw projected
  line L45 (-155.2534, -18.8832) -> (-160.4889, -24.1186) projected
  arc A105 (-176.4785, -21.5706) -> (-160.4889, -24.1186) centre (-167.5599, -17.0475) ccw projected
  line L46 (-102.4688, -28.3121) -> (-103.1912, -28.3121) projected
  arc A106 (-105.2981, -27.4478) -> (-103.1912, -28.3121) centre (-103.1912, -25.3121) ccw projected
  arc A107 (-118.1765, -13.4079) -> (-105.2981, -27.4478) centre (28.7673, 108.4524) ccw projected
  arc A108 (-120.1118, -4.3395) -> (-118.1765, -13.4079) centre (-110.479, -7.0244) ccw projected
  arc A109 (-120.1118, -4.3395) -> (-120.1128, 3.7189) centre (-134.5611, -0.3121) ccw projected
  arc A110 (-118.1829, 12.7841) -> (-120.1128, 3.7189) centre (-110.4807, 6.4063) ccw projected
  arc A111 (-97.3626, 34.2305) -> (-118.1829, 12.7841) centre (27.7313, -108.0406) ccw projected
  arc A112 (-89.0611, 30.4755) -> (-97.3626, 34.2305) centre (-94.0611, 30.4755) ccw projected
  line L47 (-89.0611, 30.4755) -> (-89.0611, -12.0997) projected
  arc A113 (-102.4688, -28.3121) -> (-89.0611, -12.0997) centre (-107.9833, -10.1012) ccw projected
  line L48 (179, 51.6879) -> (179, -0.3121)
  arc A114 (165.3495, -33.3121) -> (179, -0.3121) centre (132.2862, -0.3121) ccw
  line L49 (169.8911, -28.0259) -> (-172.1659, -28.0259)
  arc A115 (-181.2748, -0.3121) -> (-167.6243, -33.3121) centre (-134.5611, -0.3121) ccw
  line L50 (-181.2748, -0.3121) -> (-181.2748, 51.6879)
  line L51 (-181.2748, 46.4017) -> (179, 46.4017)
  line L52 (174, -0.3121) -> (174, 51.6879)
  line L53 (174, 41.4017) -> (-176.2748, 41.4017)
  line L54 (-176.2748, 51.6879) -> (-176.2748, -0.3121)
  arc A116 (-176.2748, -0.3121) -> (-160.0765, -33.3121) centre (-134.5611, -0.3121) ccw
  line L55 (-169.5485, -23.0259) -> (167.2737, -23.0259)
  arc A117 (157.8017, -33.3121) -> (174, -0.3121) centre (132.2862, -0.3121) ccw
  point P0 (0, 0)
  dimension "d121" = 5
  constraints: 16 end point, 12 point on circle, 12 point on line, 4 centre point
  measures "d121" distance between parallel lines of L48 L52
extrude "Выдавливание10" add sketch "Эскиз14" against normal blind 10 contours A117 A83 A114 L49 | L49 A114 L3 A117 | A117 A81 A114 A83 | L3 A115 L49 A116 | A117 L52 L36 A76 L48 A114 A81 | L49 A115 A105 A116 | A105 A115 A103 A116 | L52 A79 L48 A76 L36 | L52 L51 A69 L48 A79 | A115 L50 A98 L42 L54 A116 A103 | A69 L51 L48 | L52 L1 L48 A69 L51 | A69 L48 L51 | L50 A99 L54 L42 A98 | L1 L54 L51 A65 L50 | L50 A65 L51 L54 A99 | A65 L51 L50 | L50 L51 A65
sketch "Эскиз15" plane through (0, 0, 0) normal (0, 0, -1) x (-1, 0, 0)
  line L0 (-179, 48.7683) -> (-179, 51.6879) projected
  line L1 (-179.2862, 51.6879) -> (-179, 51.6879) projected
  arc A0 (-179.2862, 51.6879) -> (-184.2862, 46.6879) centre (-179.2862, 46.6879) ccw projected
  line L2 (-184.2862, -0.3121) -> (-184.2862, 46.6879) projected
  arc A1 (-184.2862, -0.3121) -> (-173.401, -32.1488) centre (-132.2862, -0.3121) ccw projected
  arc A2 (-173.401, -32.1488) -> (-171.029, -33.3121) centre (-171.029, -30.3121) ccw projected
  line L3 (-171.029, -33.3121) -> (-165.3495, -33.3121) projected
  arc A3 (-172.6737, -23.7861) -> (-165.3495, -33.3121) centre (-132.2862, -0.3121) ccw projected
  arc A4 (-174.2037, -21.5706) -> (-172.6737, -23.7861) centre (-165.2851, -17.0475) ccw projected
  arc A5 (-178.72, -7.5859) -> (-174.2037, -21.5706) centre (-132.2862, -0.3121) ccw projected
  arc A6 (-178.6766, -5.7995) -> (-178.72, -7.5859) centre (-173.7802, -6.8121) ccw projected
  arc A7 (-179, -0.3121) -> (-178.6766, -5.7995) centre (-132.2862, -0.3121) ccw projected
  line L4 (-179, -0.3121) -> (-179, 4.5205) projected
  arc A8 (-179.2862, 6.1879) -> (-179, 4.5205) centre (-174.2862, 6.1879) ccw projected
  line L5 (-179.2862, 6.1879) -> (-179.2862, 31.7702) projected
  arc A9 (-179, 33.4376) -> (-179.2862, 31.7702) centre (-174.2862, 31.7702) ccw projected
  line L6 (-179, 33.4376) -> (-179, 44.6075) projected
  arc A10 (-179, 48.7683) -> (-179, 44.6075) centre (-179.2862, 46.6879) ccw projected
  arc A11 (167.6243, -33.3121) -> (174.9485, -23.7861) centre (134.5611, -0.3121) ccw projected
  line L7 (167.6243, -33.3121) -> (173.3038, -33.3121) projected
  arc A12 (173.3038, -33.3121) -> (175.6758, -32.1488) centre (173.3038, -30.3121) ccw projected
  arc A13 (175.6758, -32.1488) -> (186.5611, -0.3121) centre (134.5611, -0.3121) ccw projected
  line L8 (186.5611, 46.6879) -> (186.5611, -0.3121) projected
  arc A14 (186.5611, 46.6879) -> (181.5611, 51.6879) centre (181.5611, 46.6879) ccw projected
  line L9 (181.2748, 51.6879) -> (181.5611, 51.6879) projected
  line L10 (181.2748, 51.6879) -> (181.2748, 48.7683) projected
  arc A15 (181.2748, 44.6075) -> (181.2748, 48.7683) centre (181.5611, 46.6879) ccw projected
  line L11 (181.2748, 44.6075) -> (181.2748, 33.4376) projected
  arc A16 (181.5611, 31.7702) -> (181.2748, 33.4376) centre (176.5611, 31.7702) ccw projected
  line L12 (181.5611, 31.7702) -> (181.5611, 6.1879) projected
  arc A17 (181.2748, 4.5205) -> (181.5611, 6.1879) centre (176.5611, 6.1879) ccw projected
  line L13 (181.2748, 4.5205) -> (181.2748, -0.3121) projected
  arc A18 (180.9514, -5.7995) -> (181.2748, -0.3121) centre (134.5611, -0.3121) ccw projected
  arc A19 (180.9948, -7.5859) -> (180.9514, -5.7995) centre (176.055, -6.8121) ccw projected
  arc A20 (176.4785, -21.5706) -> (180.9948, -7.5859) centre (134.5611, -0.3121) ccw projected
  arc A21 (174.9485, -23.7861) -> (176.4785, -21.5706) centre (167.5599, -17.0475) ccw projected
  point P0 (0, 0)
extrude "Выдавливание11" cut sketch "Эскиз15" against normal blind 10
sketch "Эскиз16" plane through (0, 0, -8) normal (0, 0, -1) x (-1, 0, 0)
  line L0 (-165.3495, -33.3121) -> (-157.8017, -33.3121) projected
  arc A0 (-174, -0.3121) -> (-157.8017, -33.3121) centre (-132.2862, -0.3121) ccw projected
  line L1 (-174, -0.3121) -> (-174, 51.6879) projected
  line L2 (-174, 51.6879) -> (-179, 51.6879) projected
  line L3 (-179, 51.6879) -> (-179, -0.3121) projected
  arc A1 (-179, -0.3121) -> (-165.3495, -33.3121) centre (-132.2862, -0.3121) ccw projected
  line L4 (181.2748, 51.6879) -> (176.2748, 51.6879) projected
  line L5 (176.2748, 51.6879) -> (176.2748, -0.3121) projected
  arc A2 (160.0765, -33.3121) -> (176.2748, -0.3121) centre (134.5611, -0.3121) ccw projected
  line L6 (160.0765, -33.3121) -> (167.6243, -33.3121) projected
  arc A3 (167.6243, -33.3121) -> (181.2748, -0.3121) centre (134.5611, -0.3121) ccw projected
  line L7 (181.2748, -0.3121) -> (181.2748, 51.6879) projected
  point P0 (0, 0)
extrude "Выдавливание12" cut sketch "Эскиз16" against normal up to surface (8 mm away)